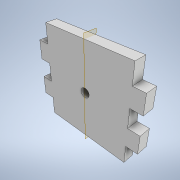
# Autodesk Inventor part: Side
Saved by Autodesk Inventor 2021.2 (Build 252289000, 289)
## iProperties
Created: 2021-03-04
Part Number: Side
Material: Generic
Document SubType Name: Modeling
Designer: 443201246
Density: 1 g/cm^3
Appearance: Default
Author: 443201246
Autodesk Inventor part; units mm, degrees
ref_plane "YZ Plane" through (0, 0, 0) normal (1, 0, 0) x (0, 1, 0)
ref_plane "XZ Plane" through (0, 0, 0) normal (0, 1, 0) x (-1, 0, 0)
ref_plane "XY Plane" through (0, 0, 0) normal (0, 0, 1) x (1, 0, 0)
sketch "Sketch1" plane through (0, 0, 0) normal (0, 0, 1) x (1, 0, 0)
  line L0 (0, 0) -> (119, 0)
  line L1 (119, 0) -> (119, 100)
  line L2 (119, 100) -> (0, 100)
  line L3 (0, 100) -> (0, 0)
  dimension "d0" = 119
  dimension "d1" = 100
  constraints: 8 end point, 2 parallel, 1 horizontal, 1 perpendicular
  measures "d0" distance of L2.end L1.end
  measures "d1" distance of L1.end L0.end
extrude "Extrusion1" add sketch "Sketch1" against normal blind 12
sketch "Sketch2" plane through (0, 0, 0) normal (0, 0, 1) x (1, 0, 0)
  line L0 (119, 0) -> (0, 0) projected
  line L1 (0, 0) -> (12, 0)
  line L2 (12, 0) -> (12, 20)
  line L3 (12, 20) -> (0, 20)
  line L4 (0, 20) -> (0, 0)
  line L5 (0, 0) -> (0, 100) projected
  line L6 (0, 40) -> (12, 40)
  line L7 (12, 40) -> (12, 60)
  line L8 (12, 60) -> (0, 60)
  line L9 (0, 60) -> (0, 40)
  line L10 (0, 100) -> (0, 0) projected
  line L11 (0, 80) -> (12, 80)
  line L12 (12, 80) -> (12, 100)
  line L13 (12, 100) -> (0, 100)
  line L14 (0, 100) -> (0, 80)
  dimension "d4" = 12
  dimension "d5" = 20
  dimension "d6" = 12
  dimension "d7" = 20
  dimension "d8" = 12
  dimension "d9" = 20
  dimension "d10" = 20
  dimension "d11" = 20
  constraints: 24 end point, 6 parallel, 3 horizontal, 3 perpendicular, 2 point on line
  measures "d4" distance of L3.end L2.end
  measures "d5" distance of L2.end L1.end
  measures "d6" distance of L8.end L7.end
  measures "d7" distance of L7.end L6.end
  measures "d8" distance of L13.end L12.end
  measures "d9" distance of L12.end L11.end
  measures "d10" distance between parallel lines of L8 L11
  measures "d11" distance between parallel lines of L3 L6
extrude "Extrusion2" cut sketch "Sketch2" against normal through all
ref_plane "Work Plane1" through (59.5, 0, 0) normal (1, 0, 0) x (0, 0, -1)
mirror "Mirror1" about plane through (59.5, 0, 0) normal (1, 0, 0) of "Extrusion2"
sketch "Sketch3" plane through (0, 0, 0) normal (0, 0, 1) x (1, 0, 0)
  circle A0 centre (59.5, 50) radius 5
  line L0 (12, 0) -> (107, 0) projected
  line L1 (0, 80) -> (0, 60) projected
  point P0 (0, 0)
  dimension "d14" = 10
  dimension "d15" = 50
  dimension "d16" = 59.5
  constraints: 1 centre point
  measures "d14" diameter of A0
  measures "d15" distance from line of L0 A0.centre
  measures "d16" distance from line of L1 A0.centre
extrude "Extrusion3" cut sketch "Sketch3" against normal through all
body "Solid1"
